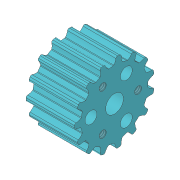
# Autodesk Inventor part: TIMING_BELT_P15
Saved by Autodesk Inventor 2019.4 (Build 234330000, 330)
## iProperties
Created: 2019-11-09
Part Number: TIMING_BELT_P15
Material: 一般
Document SubType Name: Modeling
Designer: y6tada
Density: 1 g/cm^3
Appearance: くすんだ青
Author: y6tada
Autodesk Inventor part; units mm, degrees
ref_plane "YZ Plane" through (0, 0, 0) normal (1, 0, 0) x (0, 1, 0)
ref_plane "XZ Plane" through (0, 0, 0) normal (0, 1, 0) x (-1, 0, 0)
ref_plane "XY Plane" through (0, 0, 0) normal (0, 0, 1) x (1, 0, 0)
sketch "スケッチ1" plane through (0, 0, 0) normal (1, 0, 0) x (0, 1, 0)
  arc A0 (0.9732, -6.7098) -> (0, -6.78) centre (0, 0) ccw construction
  line L0 (0, 0) -> (0, -15.5638) construction
  line L1 (0.975, -7.034) -> (-0.975, -7.034) construction
  arc A1 (0.9732, -6.7098) -> (0.437, -5.6531) centre (-0.975, -7.034) ccw
  arc A2 (-0.437, -5.6531) -> (0.437, -5.6531) centre (0, 0) ccw
  arc A3 (-0.437, -5.6531) -> (-0.9732, -6.7098) centre (0.975, -7.034) ccw
  circle A4 centre (0, 0) radius 14.32 construction
  line L2 (0, -6.78) -> (0.975, -6.78) construction
  circle A5 centre (0, 0) radius 7.16 construction
  line L3 (1.4096, -6.6318) -> (0, 0)
  line L4 (0, 0) -> (-1.4096, -6.6318)
  arc A6 (-1.4096, -6.6318) -> (-0.9732, -6.7098) centre (0, 0) ccw
  arc A7 (0.9732, -6.7098) -> (1.4096, -6.6318) centre (0, 0) ccw
  dimension "d2" = 1.95
  dimension "d3" = 1.975
  dimension "d4" = 1.11
  dimension "d8" = 0.254
  dimension "d10" = 13.56
  dimension "d11" = 14.32
  dimension "d12" = 24
  constraints: 14 point on circle, 10 end point, 8 centre point, 4 symmetric about line, 3 coincident, 1 concentric, 1 horizontal, 1 perpendicular, 1 point on line, 1 tangent, 1 vertical, 1 other
  measures "d2" distance of L1.start L1.end
  measures "d3" radius of A1
  measures "d4" radial gap between concentric circles of A0 A2
  measures "d8" distance between parallel lines of L1 L2
  measures "d10" diameter of A0
  measures "d11" diameter of A5
  measures "d12" angle of L4 L3
extrude "押し出し1" add sketch "スケッチ1" along normal mid plane 8.2
fillet "フィレット1" radius 0.15 2 edges at (0, 0.437, -5.6531) (0, -0.437, -5.6531)
fillet "フィレット2" radius 0.28 2 edges at (0, 0.9732, -6.7098) (0, -0.9732, -6.7098)
pattern_circular "円形状パターン1" count 15 over 360 about axis through (-10, 0, 0) along (1, 0, 0)
sketch "スケッチ2" plane through (4.1, 0, 0) normal (1, 0, 0) x (0, 0, -1)
  point P0 (0, 0)
  point P1 (0, 0)
  constraints: 1 coincident
hole "穴1" at (4.1, 0, 0) direction (-1, 0, 0) diameter 3 end through all
sketch "スケッチ3" plane through (4.1, 0, 0) normal (1, 0, 0) x (0, 0, -1)
  circle A0 centre (0, 0) radius 4 construction
  circle A1 centre (4, 0) radius 1.5 construction
  line L0 (0, 0) -> (4, 0) construction
  point P0 (2, 3.4641)
  point P1 (-2, 3.4641)
  point P2 (-4, 0)
  point P3 (-2, -3.4641)
  point P4 (2, -3.4641)
  dimension "d27" = 8
  dimension "d28" = 3
  dimension "d31" = 360
  constraints: 2 coincident, 2 end point, 1 centre point, 1 horizontal, 1 horizontal alignment, 9 other
  measures "d28" diameter of A1
hole "穴2" at (4.1, 0, -4) at (4.1, 3.4641, 2) at (4.1, -3.4641, 2) direction (-1, 0, 0) diameter 1.183 end through all thread size "M1.4x0.3" class "6H" standard "ISO Metric profile"
hole "穴3" at (4.1, 3.4641, -2) at (4.1, 0, 4) at (4.1, -3.4641, -2) direction (-1, 0, 0) diameter 2 end through all
